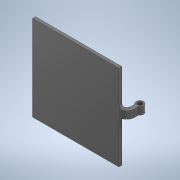
# Autodesk Inventor part: TapasContenedor
Saved by Autodesk Inventor 2020.3 (Build 243373000, 373)
## iProperties
Created: 2020-11-08
Part Number: TapasContenedor
Material: ABS Plastic
Document SubType Name: Modeling
Designer: juanp
Density: 1.06 g/cm^3
Appearance: Smooth - White
Mass: 26.2392 g
Surface Area: 177.889 cm^2
Volume: 24.7539 cm^3
Author: juanp
Autodesk Inventor part; units mm, degrees
ref_plane "YZ Plane" through (0, 0, 0) normal (1, 0, 0) x (0, 1, 0)
sketch "Sketch1" plane through (0, 0, 0) normal (0, 0, 1) x (1, 0, 0)
  line L0 (0, 0) -> (90, 0)
  line L1 (90, 0) -> (90, 89.197)
  line L2 (90, 89.197) -> (0, 89.197)
  line L3 (0, 89.197) -> (0, 0)
  dimension "d0" = 90
  dimension "d1" = 89.197
  constraints: 8 end point, 2 parallel, 1 horizontal, 1 perpendicular
  measures "d0" distance of L2.end L1.end
  measures "d1" distance of L1.end L0.end
extrude "Extrusion1" add sketch "Sketch1" along normal blind 3
ref_plane "Work Plane1" through (0, 44.5985, 0) normal (0, -1, 0) x (1, 0, 0)
ref_plane "Work Plane2" through (0, 47.446, 0) normal (0, 1, 0) x (1, 0, 0)
sketch "Sketch12" plane through (0, 47.446, 0) normal (0, 1, 0) x (1, 0, 0)
  line L0 (90, 0) -> (96.1, 0) construction
  line L1 (96.1, 0) -> (96.1, 12.7) construction
  line L2 (96.1, 12.7) -> (90, 12.7) construction
  line L3 (90, 12.7) -> (90, 0) construction
  line L4 (90, 0) -> (0, 0) projected
  line L5 (90, -3) -> (0, -3) projected
  circle A0 centre (96.1, 12.7) radius 3.9
  circle A1 centre (96.1, 12.7) radius 2.4
  line L6 (90, 0) -> (90, -3) projected
  line L7 (90, -3) -> (93.6569, -3)
  line L8 (90, 0) -> (91, 0)
  line L9 (98.1, 9.3519) -> (98.1, 1.4431)
  line L10 (94.1, 9.3519) -> (94.1, 3.1)
  line L11 (98.1, 4.1404) -> (96.1, 4.1404)
  line L12 (96.1, 7.8099) -> (94.1, 7.8099)
  line L13 (98.1, 1.4431) -> (93.6569, -3)
  line L14 (94.1, 3.1) -> (91, 0)
  dimension "d37" = 12.7
  dimension "d38" = 6.1
  dimension "d40" = 4.8
  dimension "d41" = 1.5
  dimension "d45" = 1
  dimension "d46" = 4
  dimension "d47" = 45
  dimension "d48" = 4
  constraints: 26 end point, 5 point on line, 4 parallel, 3 perpendicular, 2 centre point, 2 coincident, 2 horizontal, 2 point on circle, 2 vertical
  measures "d37" distance of L2.end L0.start
  measures "d38" distance of L1.end L2.end
  measures "d40" diameter of A1
  measures "d41" radial gap between concentric circles of A1 A0
  measures "d45" distance of L0.start L8.end
  measures "d46" distance between parallel lines of L9 L10
  measures "d47" angle of L0 L14
  measures "d48" distance between parallel lines of L13 L14
extrude "Extrusion9" add sketch "Sketch12" against normal blind 2.7
sketch "Sketch13" plane through (0, 47.446, 0) normal (0, 1, 0) x (1, 0, 0)
  line L0 (94.1, 9.3519) -> (94.1, 3.1) projected
  line L1 (94.1, 3.1) -> (91, 0) projected
  line L2 (91, 0) -> (90, 0) projected
  line L3 (90, -3) -> (90, 0) projected
  line L4 (90, -3) -> (93.6569, -3) projected
  line L5 (93.6569, -3) -> (98.1, 1.4431) projected
  line L6 (98.1, 1.4431) -> (98.1, 9.3519) projected
  arc A0 (98.1, 9.3519) -> (94.1, 9.3519) centre (96.1, 12.7) ccw projected
  circle A1 centre (96.1, 12.7) radius 2.4 projected
  circle A2 centre (96.1, 12.7) radius 1
  point P0 (0, 0)
  dimension "d51" = 2
  constraints: 1 centre point, 1 coincident
  measures "d51" diameter of A2
extrude "Extrusion10" add sketch "Sketch13" along normal blind 1 contours A0 L6 L5 L4 L3 L2 L1 L0 | A1
extrude "Extrusion11" add sketch "Sketch12" along normal blind 5
fillet "Fillet5" radius 4 2 edges at (90, 52.446, 1.5) (90, 44.746, 1.5)
fillet "Fillet6" radius 8 3 edges at (94.1, 48.596, -3.1) (93.6569, 48.596, 3) (98.1, 48.596, -1.4431)
body "Solid1"
